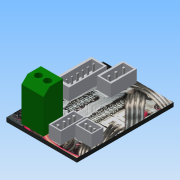
# Autodesk Inventor part: разводка
Saved by Autodesk Inventor 2017 (Build 210142000, 142)
## iProperties
Part Number: разводка
Material: Типовые
Document SubType Name: Modeling
Designer: Max
Mass: 6.97711 g
Surface Area: 88.2205 cm^2
Volume: 6.97711 cm^3
Density: 1 g/cm^3
Appearance: Оружейный металл — полированный
Author: Max
Autodesk Inventor part; units mm, degrees
ref_plane "YZ Plane" through (0, 0, 0) normal (1, 0, 0) x (0, 1, 0)
ref_plane "XZ Plane" through (0, 0, 0) normal (0, 1, 0) x (-1, 0, 0)
ref_plane "XY Plane" through (0, 0, 0) normal (0, 0, 1) x (1, 0, 0)
sketch "Эскиз1" plane through (0, 0, 0) normal (0, 0, 1) x (1, 0, 0)
  line L0 (-172.6613, 135.7054) -> (-137.6613, 135.7054)
  line L1 (-137.6613, 135.7054) -> (-137.6613, 87.7054)
  line L2 (-137.6613, 87.7054) -> (-172.6613, 87.7054)
  line L3 (-172.6613, 87.7054) -> (-172.6613, 135.7054)
  point P0 (0, 0)
  dimension "d13" = 48
  dimension "d14" = 35
  constraints: 8 end point, 2 parallel, 1 horizontal, 1 perpendicular
  measures "d13" distance between parallel lines of L2 L0
  measures "d14" distance between parallel lines of L1 L3
extrude "Выдавливание1" add sketch "Эскиз1" along normal blind 2
sketch "Эскиз2" plane through (0, 0, 2) normal (0, 0, 1) x (1, 0, 0)
  line L0 (-189.4202, 27.633) -> (-189.4202, 179.0614) construction
  line L1 (-189.4202, 179.0614) -> (-119.4698, 179.0614) construction
  line L2 (-119.4698, 179.0614) -> (-119.4698, 27.633) construction
  line L3 (-119.4698, 27.633) -> (-189.4202, 27.633) construction
  line L4 (-137.6613, 135.7054) -> (-172.6613, 135.7054) projected
  line L5 (-172.6613, 135.7054) -> (-172.6613, 87.7054) projected
  line L6 (-172.6613, 87.7054) -> (-137.6613, 87.7054) projected
  line L7 (-137.6613, 87.7054) -> (-137.6613, 135.7054) projected
  point P0 (0, 0)
  constraints: 2 other
decal "Маркировка1"
sketch "Эскиз3" plane through (0, 0, 2) normal (0, 0, 1) x (1, 0, 0)
  line L0 (-153.1945, 89.2305) -> (-147.0972, 89.2305)
  line L1 (-147.0972, 89.2305) -> (-147.0972, 101.5189)
  line L2 (-147.0972, 101.5189) -> (-153.1945, 101.5189)
  line L3 (-153.1945, 101.5189) -> (-153.1945, 89.2305)
  line L4 (-152.4669, 89.7529) -> (-147.5681, 89.7529)
  line L5 (-147.5681, 89.7529) -> (-147.5681, 100.9856)
  line L6 (-147.5681, 100.9856) -> (-152.4669, 100.9856)
  line L7 (-152.4669, 100.9856) -> (-152.4669, 89.7529)
  line L8 (-146.4299, 95.6909) -> (-138.3147, 95.6909)
  line L9 (-138.3147, 95.6909) -> (-138.3147, 101.5189)
  line L10 (-138.3147, 101.5189) -> (-146.4299, 101.5189)
  line L11 (-146.4299, 101.5189) -> (-146.4299, 95.6909)
  line L12 (-145.6877, 96.2352) -> (-138.76, 96.2352)
  line L13 (-138.76, 96.2352) -> (-138.76, 100.9856)
  line L14 (-138.76, 100.9856) -> (-145.6877, 100.9856)
  line L15 (-145.6877, 100.9856) -> (-145.6877, 96.2352)
  line L16 (-151.0319, 90.8415) -> (-150.1459, 90.8415)
  line L17 (-150.1459, 90.8415) -> (-150.1459, 91.6333)
  line L18 (-150.1459, 91.6333) -> (-151.0319, 91.6333)
  line L19 (-151.0319, 91.6333) -> (-151.0319, 90.8415)
  line L20 (-151.0319, 93.9095) -> (-150.1459, 93.9095)
  line L21 (-150.1459, 93.9095) -> (-150.1459, 94.6518)
  line L22 (-150.1459, 94.6518) -> (-151.0319, 94.6518)
  line L23 (-151.0319, 94.6518) -> (-151.0319, 93.9095)
  line L24 (-151.0319, 96.2352) -> (-150.1459, 96.2352)
  line L25 (-150.1459, 96.2352) -> (-150.1459, 97.027)
  line L26 (-150.1459, 97.027) -> (-151.0319, 97.027)
  line L27 (-151.0319, 97.027) -> (-151.0319, 96.2352)
  line L28 (-151.0319, 98.6104) -> (-150.1459, 98.6104)
  line L29 (-150.1459, 98.6104) -> (-150.1459, 99.5506)
  line L30 (-150.1459, 99.5506) -> (-151.0319, 99.5506)
  line L31 (-151.0319, 99.5506) -> (-151.0319, 98.6104)
  line L32 (-144.6485, 98.264) -> (-143.7578, 98.264)
  line L33 (-143.7578, 98.264) -> (-143.7578, 99.0805)
  line L34 (-143.7578, 99.0805) -> (-144.6485, 99.0805)
  line L35 (-144.6485, 99.0805) -> (-144.6485, 98.264)
  line L36 (-142.3723, 98.264) -> (-141.5311, 98.264)
  line L37 (-141.5311, 98.264) -> (-141.5311, 99.0805)
  line L38 (-141.5311, 99.0805) -> (-142.3723, 99.0805)
  line L39 (-142.3723, 99.0805) -> (-142.3723, 98.264)
  line L40 (-140.294, 98.264) -> (-139.6507, 98.264)
  line L41 (-139.6507, 98.264) -> (-139.6507, 99.0805)
  line L42 (-139.6507, 99.0805) -> (-140.294, 99.0805)
  line L43 (-140.294, 99.0805) -> (-140.294, 98.264)
  line L44 (-171.7271, 110.0545) -> (-163.9092, 110.0545)
  line L45 (-163.9092, 110.0545) -> (-163.9092, 128.8628)
  line L46 (-163.9092, 128.8628) -> (-171.7271, 128.8628)
  line L47 (-171.7271, 128.8628) -> (-171.7271, 110.0545)
  line L48 (-170.552, 111.3682) -> (-164.5795, 111.3682)
  line L49 (-164.5795, 111.3682) -> (-164.5795, 127.9697)
  line L50 (-164.5795, 127.9697) -> (-170.552, 127.9697)
  line L51 (-170.552, 127.9697) -> (-170.552, 111.3682)
  line L52 (-168.2693, 112.635) -> (-167.8181, 112.635)
  line L53 (-167.8181, 112.635) -> (-167.8181, 113.2224)
  line L54 (-167.8181, 113.2224) -> (-168.2693, 113.2224)
  line L55 (-168.2693, 113.2224) -> (-168.2693, 112.635)
  line L56 (-168.2693, 115.2471) -> (-167.8181, 115.2471)
  line L57 (-167.8181, 115.2471) -> (-167.8181, 115.9603)
  line L58 (-167.8181, 115.9603) -> (-168.2693, 115.9603)
  line L59 (-168.2693, 115.9603) -> (-168.2693, 115.2471)
  line L60 (-168.2693, 117.8624) -> (-167.8181, 117.8624)
  line L61 (-167.8181, 117.8624) -> (-167.8181, 118.7985)
  line L62 (-167.8181, 118.7985) -> (-168.2693, 118.7985)
  line L63 (-168.2693, 118.7985) -> (-168.2693, 117.8624)
  line L64 (-168.2693, 120.5817) -> (-167.8181, 120.5817)
  line L65 (-167.8181, 120.5817) -> (-167.8181, 121.2949)
  line L66 (-167.8181, 121.2949) -> (-168.2693, 121.2949)
  line L67 (-168.2693, 121.2949) -> (-168.2693, 120.5817)
  line L68 (-168.2693, 123.1748) -> (-167.8181, 123.1748)
  line L69 (-167.8181, 123.1748) -> (-167.8181, 123.9393)
  line L70 (-167.8181, 123.9393) -> (-168.2693, 123.9393)
  line L71 (-168.2693, 123.9393) -> (-168.2693, 123.1748)
  line L72 (-168.2693, 125.9405) -> (-167.8181, 125.9405)
  line L73 (-167.8181, 125.9405) -> (-167.8181, 126.705)
  line L74 (-167.8181, 126.705) -> (-168.2693, 126.705)
  line L75 (-168.2693, 126.705) -> (-168.2693, 125.9405)
  line L76 (-162.1006, 122.0648) -> (-155.1613, 122.0648)
  line L77 (-155.1613, 122.0648) -> (-155.1613, 134.9002)
  line L78 (-155.1613, 134.9002) -> (-162.1006, 134.9002)
  line L79 (-162.1006, 134.9002) -> (-162.1006, 122.0648)
  line L80 (-161.1331, 122.7743) -> (-155.9732, 122.7743)
  line L81 (-155.9732, 122.7743) -> (-155.9732, 134.1907)
  line L82 (-155.9732, 134.1907) -> (-161.1331, 134.1907)
  line L83 (-161.1331, 134.1907) -> (-161.1331, 122.7743)
  line L84 (-159.3916, 124.5158) -> (-158.631, 124.5158)
  line L85 (-158.631, 124.5158) -> (-158.631, 125.4188)
  line L86 (-158.631, 125.4188) -> (-159.3916, 125.4188)
  line L87 (-159.3916, 125.4188) -> (-159.3916, 124.5158)
  line L88 (-159.3916, 127.9697) -> (-158.631, 127.9697)
  line L89 (-158.631, 127.9697) -> (-158.631, 128.8628)
  line L90 (-158.631, 128.8628) -> (-159.3916, 128.8628)
  line L91 (-159.3916, 128.8628) -> (-159.3916, 127.9697)
  line L92 (-159.3916, 131.8042) -> (-158.631, 131.8042)
  line L93 (-158.631, 131.8042) -> (-158.631, 132.6427)
  line L94 (-158.631, 132.6427) -> (-159.3916, 132.6427)
  line L95 (-159.3916, 132.6427) -> (-159.3916, 131.8042)
  line L96 (-166.0996, 88.6541) -> (-155.1613, 88.6541)
  line L97 (-155.1613, 88.6541) -> (-155.1613, 98.264)
  line L98 (-155.1613, 98.264) -> (-166.0996, 98.264)
  line L99 (-166.0996, 98.264) -> (-166.0996, 88.6541)
  circle A0 centre (-162.7529, 93.6775) radius 1.6681
  circle A1 centre (-158.2242, 93.6775) radius 1.7261
  point P0 (0, 0)
  constraints: 200 end point, 50 parallel, 25 horizontal, 25 perpendicular, 21 point on line, 2 centre point
extrude "Выдавливание2" add sketch "Эскиз3" along normal blind 20 contours L99 L98 L97 L96
chamfer "Фаска1" distance 3 angle 45 1 edges at (-160.6304, 88.6541, 22)
extrude "Выдавливание3" add sketch "Эскиз3" along normal blind 1 contours L7 L6 L5 L4 | L15 L14 L13 L12 | L51 L50 L49 L48 | L83 L82 L81 L80
extrude "Выдавливание4" add sketch "Эскиз3" along normal blind 6 contours L3 L2 L1 L0 | L11 L10 L9 L8 | L19 L18 L17 L16 | L23 L22 L21 L20 | L27 L26 L25 L24 | L31 L30 L29 L28 | L35 L34 L33 L32 | L39 L38 L37 L36 | L43 L42 L41 L40 | L47 L46 L45 L44 | L55 L54 L53 L52 | L59 L58 L57 L56 | L63 L62 L61 L60 | L67 L66 L65 L64 | L71 L70 L69 L68 | L75 L74 L73 L72 | L79 L78 L77 L76 | L87 L86 L85 L84 | L91 L90 L89 L88 | L95 L94 L93 L92
sketch "Эскиз4" plane through (0, 0, 0) normal (0, 0, -1) x (-1, 0, 0)
  circle A0 centre (17.5613, 127.4954) radius 1.5 projected
  circle A1 centre (-13.4387, 158.4954) radius 1.5 projected
  circle A2 centre (17.5613, 158.4954) radius 1.5 projected
  circle A3 centre (-13.4387, 127.4954) radius 1.5 projected
  line L0 (91.0613, 108.9954) -> (91.0613, 96.9954) projected
  line L1 (91.0613, 96.9954) -> (71.0613, 96.9954) projected
  line L2 (71.0613, 96.9954) -> (71.0613, 108.9954) projected
  line L3 (71.0613, 108.9954) -> (91.0613, 108.9954) projected
  line L4 (170.6613, 127.5954) -> (170.6613, 101.5954) projected
  line L5 (170.6613, 101.5954) -> (142.6613, 101.5954) projected
  line L6 (142.6613, 101.5954) -> (142.6613, 127.5954) projected
  line L7 (142.6613, 127.5954) -> (170.6613, 127.5954) projected
  circle A4 centre (-90.4387, 142.9954) radius 6 projected
  circle A5 centre (-101.4387, 142.9954) radius 1.5 projected
  circle A6 centre (105.5613, 142.9954) radius 1.5 projected
  circle A7 centre (83.5613, 142.9954) radius 1.5 projected
  circle A8 centre (-79.4387, 142.9954) radius 1.5 projected
  circle A9 centre (94.5613, 142.9954) radius 6 projected
  circle A10 centre (2.0613, 142.9954) radius 11.5 projected
  line L8 (-135.5937, -165.0046) -> (-186.9387, -165.0046) projected
  line L9 (-104.3113, -105.8851) -> (-135.5937, -165.0046) projected
  line L10 (108.4339, -105.8851) -> (-104.3113, -105.8851) projected
  line L11 (139.7163, -165.0046) -> (108.4339, -105.8851) projected
  line L12 (191.0613, -165.0046) -> (139.7163, -165.0046) projected
  line L13 (191.0613, 166.9954) -> (191.0613, -165.0046) projected
  line L14 (-186.9387, 166.9954) -> (191.0613, 166.9954) projected
  line L15 (-186.9387, -165.0046) -> (-186.9387, 166.9954) projected
  line L16 (146.8954, 125.9954) -> (152.6047, 125.9954)
  line L17 (152.6047, 125.9954) -> (152.6047, 102.9954)
  line L18 (152.6047, 102.9954) -> (146.8954, 102.9954)
  line L19 (146.8954, 102.9954) -> (146.8954, 125.9954)
  line L20 (147.4728, 125.3387) -> (152.1557, 125.3387)
  line L21 (152.1557, 125.3387) -> (152.1557, 103.4637)
  line L22 (152.1557, 103.4637) -> (147.4728, 103.4637)
  line L23 (147.4728, 103.4637) -> (147.4728, 125.3387)
  line L24 (148.38, 124.4695) -> (149.0229, 124.4695)
  line L25 (149.0229, 124.4695) -> (149.0229, 124.0295)
  line L26 (149.0229, 124.0295) -> (148.38, 124.0295)
  line L27 (148.38, 124.0295) -> (148.38, 124.4695)
  line L28 (150.4781, 124.4695) -> (151.1549, 124.4695)
  line L29 (151.1549, 124.4695) -> (151.1549, 124.0295)
  line L30 (151.1549, 124.0295) -> (150.4781, 124.0295)
  line L31 (150.4781, 124.0295) -> (150.4781, 124.4695)
  line L32 (148.38, 121.2595) -> (148.38, 121.6995)
  line L33 (148.38, 121.6995) -> (149.0229, 121.6995)
  line L34 (149.0229, 121.6995) -> (149.0229, 121.2595)
  line L35 (149.0229, 121.2595) -> (148.38, 121.2595)
  line L36 (150.4781, 121.2595) -> (150.4781, 121.6995)
  line L37 (150.4781, 121.6995) -> (151.1549, 121.6995)
  line L38 (151.1549, 121.6995) -> (151.1549, 121.2595)
  line L39 (151.1549, 121.2595) -> (150.4781, 121.2595)
  line L40 (148.38, 118.4895) -> (148.38, 118.9295)
  line L41 (148.38, 118.9295) -> (149.0229, 118.9295)
  line L42 (149.0229, 118.9295) -> (149.0229, 118.4895)
  line L43 (149.0229, 118.4895) -> (148.38, 118.4895)
  line L44 (150.4781, 118.4895) -> (150.4781, 118.9295)
  line L45 (150.4781, 118.9295) -> (151.1549, 118.9295)
  line L46 (151.1549, 118.9295) -> (151.1549, 118.4895)
  line L47 (151.1549, 118.4895) -> (150.4781, 118.4895)
  line L48 (148.38, 115.7195) -> (148.38, 116.1595)
  line L49 (148.38, 116.1595) -> (149.0229, 116.1595)
  line L50 (149.0229, 116.1595) -> (149.0229, 115.7195)
  line L51 (149.0229, 115.7195) -> (148.38, 115.7195)
  line L52 (150.4781, 115.7195) -> (150.4781, 116.1595)
  line L53 (150.4781, 116.1595) -> (151.1549, 116.1595)
  line L54 (151.1549, 116.1595) -> (151.1549, 115.7195)
  line L55 (151.1549, 115.7195) -> (150.4781, 115.7195)
  line L56 (148.38, 112.9495) -> (148.38, 113.3895)
  line L57 (148.38, 113.3895) -> (149.0229, 113.3895)
  line L58 (149.0229, 113.3895) -> (149.0229, 112.9495)
  line L59 (149.0229, 112.9495) -> (148.38, 112.9495)
  line L60 (150.4781, 112.9495) -> (150.4781, 113.3895)
  line L61 (150.4781, 113.3895) -> (151.1549, 113.3895)
  line L62 (151.1549, 113.3895) -> (151.1549, 112.9495)
  line L63 (151.1549, 112.9495) -> (150.4781, 112.9495)
  line L64 (148.38, 110.1795) -> (148.38, 110.6195)
  line L65 (148.38, 110.6195) -> (149.0229, 110.6195)
  line L66 (149.0229, 110.6195) -> (149.0229, 110.1795)
  line L67 (149.0229, 110.1795) -> (148.38, 110.1795)
  line L68 (150.4781, 110.1795) -> (150.4781, 110.6195)
  line L69 (150.4781, 110.6195) -> (151.1549, 110.6195)
  line L70 (151.1549, 110.6195) -> (151.1549, 110.1795)
  line L71 (151.1549, 110.1795) -> (150.4781, 110.1795)
  line L72 (148.38, 107.4095) -> (148.38, 107.8495)
  line L73 (148.38, 107.8495) -> (149.0229, 107.8495)
  line L74 (149.0229, 107.8495) -> (149.0229, 107.4095)
  line L75 (149.0229, 107.4095) -> (148.38, 107.4095)
  line L76 (150.4781, 107.4095) -> (150.4781, 107.8495)
  line L77 (150.4781, 107.8495) -> (151.1549, 107.8495)
  line L78 (151.1549, 107.8495) -> (151.1549, 107.4095)
  line L79 (151.1549, 107.4095) -> (150.4781, 107.4095)
  line L80 (148.38, 104.6395) -> (148.38, 105.0795)
  line L81 (148.38, 105.0795) -> (149.0229, 105.0795)
  line L82 (149.0229, 105.0795) -> (149.0229, 104.6395)
  line L83 (149.0229, 104.6395) -> (148.38, 104.6395)
  line L84 (150.4781, 104.6395) -> (150.4781, 105.0795)
  line L85 (150.4781, 105.0795) -> (151.1549, 105.0795)
  line L86 (151.1549, 105.0795) -> (151.1549, 104.6395)
  line L87 (151.1549, 104.6395) -> (150.4781, 104.6395)
  line L88 (155.6162, 116.1595) -> (163.0382, 116.1595)
  line L89 (163.0382, 116.1595) -> (163.0382, 103.4637)
  line L90 (163.0382, 103.4637) -> (155.6162, 103.4637)
  line L91 (155.6162, 103.4637) -> (155.6162, 116.1595)
  line L92 (146.8954, 119.3985) -> (144.9162, 119.3985)
  line L93 (144.9162, 119.3985) -> (144.9162, 108.9954)
  line L94 (144.9162, 108.9954) -> (146.8954, 108.9954)
  line L95 (146.8954, 108.9954) -> (146.8954, 119.3985)
  line L96 (146.8954, 118.4895) -> (145.9058, 118.4895)
  line L97 (145.9058, 118.4895) -> (145.9058, 109.8116)
  line L98 (145.9058, 109.8116) -> (146.8954, 109.8116)
  line L99 (146.8954, 109.8116) -> (146.8954, 118.4895)
  line L100 (156.6613, 115.1309) -> (162.296, 115.1309)
  line L101 (162.296, 115.1309) -> (162.296, 104.1835)
  line L102 (162.296, 104.1835) -> (156.6613, 104.1835)
  line L103 (156.6613, 104.1835) -> (156.6613, 115.1309)
  line L104 (158.585, 113.832) -> (159.3272, 113.832)
  line L105 (159.3272, 113.832) -> (159.3272, 112.9495)
  line L106 (159.3272, 112.9495) -> (158.585, 112.9495)
  line L107 (158.585, 112.9495) -> (158.585, 113.832)
  line L108 (158.585, 111.2344) -> (159.3272, 111.2344)
  line L109 (159.3272, 111.2344) -> (159.3272, 110.6195)
  line L110 (159.3272, 110.6195) -> (158.585, 110.6195)
  line L111 (158.585, 110.6195) -> (158.585, 111.2344)
  line L112 (158.585, 108.9954) -> (159.3272, 108.9954)
  line L113 (159.3272, 108.9954) -> (159.3272, 107.8495)
  line L114 (159.3272, 107.8495) -> (158.585, 107.8495)
  line L115 (158.585, 107.8495) -> (158.585, 108.9954)
  line L116 (158.585, 106.3482) -> (159.3272, 106.3482)
  line L117 (159.3272, 106.3482) -> (159.3272, 105.0795)
  line L118 (159.3272, 105.0795) -> (158.585, 105.0795)
  line L119 (158.585, 105.0795) -> (158.585, 106.3482)
  line L120 (164.2133, 112.595) -> (169.5324, 112.595)
  line L121 (169.5324, 112.595) -> (169.5324, 103.4637)
  line L122 (169.5324, 103.4637) -> (164.2133, 103.4637)
  line L123 (164.2133, 103.4637) -> (164.2133, 112.595)
  line L124 (164.5795, 127.9697) -> (164.5795, 111.3682) projected
  line L125 (164.5795, 115.1309) -> (169.5324, 115.1309)
  line L126 (169.5324, 115.1309) -> (169.5324, 125.3387)
  line L127 (169.5324, 125.3387) -> (164.5795, 125.3387)
  line L128 (164.5795, 125.3387) -> (164.5795, 115.1309)
  line L129 (165.3888, 124.0295) -> (168.9139, 124.0295)
  line L130 (168.9139, 124.0295) -> (168.9139, 116.1595)
  line L131 (168.9139, 116.1595) -> (165.3888, 116.1595)
  line L132 (165.3888, 116.1595) -> (165.3888, 124.0295)
  line L133 (164.9555, 111.7292) -> (168.9139, 111.7292)
  line L134 (168.9139, 111.7292) -> (168.9139, 104.1835)
  line L135 (168.9139, 104.1835) -> (164.9555, 104.1835)
  line L136 (164.9555, 104.1835) -> (164.9555, 111.7292)
  line L137 (163.9092, 110.0545) -> (171.7271, 110.0545) projected
  line L138 (166.3781, 110.0545) -> (166.9347, 110.0545)
  line L139 (166.9347, 110.0545) -> (166.9347, 109.2383)
  line L140 (166.9347, 109.2383) -> (166.3781, 109.2383)
  line L141 (166.3781, 109.2383) -> (166.3781, 110.0545)
  line L142 (166.3781, 106.843) -> (166.9966, 106.843)
  line L143 (166.9966, 106.843) -> (166.9966, 105.7138)
  line L144 (166.9966, 105.7138) -> (166.3781, 105.7138)
  line L145 (166.3781, 105.7138) -> (166.3781, 106.843)
  line L146 (166.6564, 122.7365) -> (167.3619, 122.7365)
  line L147 (167.3619, 122.7365) -> (167.3619, 121.9552)
  line L148 (167.3619, 121.9552) -> (166.6564, 121.9552)
  line L149 (166.6564, 121.9552) -> (166.6564, 122.7365)
  line L150 (166.6564, 120.4707) -> (167.3619, 120.4707)
  line L151 (167.3619, 120.4707) -> (167.3619, 119.8978)
  line L152 (167.3619, 119.8978) -> (166.6564, 119.8978)
  line L153 (166.6564, 119.8978) -> (166.6564, 120.4707)
  line L154 (166.6564, 118.3352) -> (167.3619, 118.3352)
  line L155 (167.3619, 118.3352) -> (167.3619, 117.7362)
  line L156 (167.3619, 117.7362) -> (166.6564, 117.7362)
  line L157 (166.6564, 117.7362) -> (166.6564, 118.3352)
  point P0 (0, 0)
  dimension "d34" = 2.77
  constraints: 280 end point, 42 parallel, 33 point on line, 21 horizontal, 21 perpendicular, 1 vertical, 112 other
  measures "d34" distance of L24.start L32.end
extrude "Выдавливание5" add sketch "Эскиз4" along normal blind 1 contours L137 L136 L133 L134 | L134 L135 L136 L137 L141 L140 L139 | L20 L21 L22 L23 | L100 L101 L102 L103 | L129 L130 L131 L132
extrude "Выдавливание6" add sketch "Эскиз4" along normal blind 6 contours L137 L134 L133 L136 L123 L120 L121 | L121 L122 L123 L137 L136 L135 L134 | L127 L126 L125 L124 | L139 L140 L141 L137 | L16 L17 L18 L19 | L19 L96 L97 L98 L94 L93 L92 | L24 L25 L26 L27 | L28 L29 L30 L31 | L32 L33 L34 L35 | L36 L37 L38 L39 | L40 L41 L42 L43 | L44 L45 L46 L47 | L48 L49 L50 L51 | L52 L53 L54 L55 | L56 L57 L58 L59 | L60 L61 L62 L63 | L64 L65 L66 L67 | L68 L69 L70 L71 | L72 L73 L74 L75 | L76 L77 L78 L79 | L80 L81 L82 L83 | L84 L85 L86 L87 | L88 L89 L90 L91 | L104 L105 L106 L107 | L108 L109 L110 L111 | L112 L113 L114 L115 | L116 L117 L118 L119 | L142 L143 L144 L145 | L146 L147 L148 L149 | L150 L151 L152 L153 | L154 L155 L156 L157
